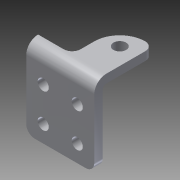
# Autodesk Inventor part: Clamp Piston Right Mount
Saved by Autodesk Inventor 2014 (Build 180170000, 170)
## iProperties
Created: 2014-02-22
Part Number: Clamp Piston Right Mount
Material: Aluminum 6061
Document SubType Name: Sheet Metal
Designer: Michael
Density: 1 g/cm^3
Sheet Metal Rule: Default
Appearance: Aluminum - Flat
Author: Michael
Autodesk Inventor part; units mm, degrees
ref_plane "YZ Plane" through (0, 0, 0) normal (1, 0, 0) x (0, 1, 0)
ref_plane "XZ Plane" through (0, 0, 0) normal (0, 1, 0) x (-1, 0, 0)
ref_plane "XY Plane" through (0, 0, 0) normal (0, 0, 1) x (1, 0, 0)
sketch "Sketch1" plane through (0, 0, 0) normal (0, 0, 1) x (1, 0, 0)
  line L0 (0, 0) -> (25.4, 0)
  line L1 (25.4, 0) -> (25.4, 25.4)
  line L2 (25.4, 25.4) -> (0, 25.4)
  line L3 (0, 25.4) -> (0, 0)
  circle A0 centre (6.35, 19.05) radius 2.0701
  circle A1 centre (19.05, 19.05) radius 2.0701
  circle A2 centre (6.35, 6.35) radius 2.0701
  circle A3 centre (19.05, 6.35) radius 2.0701
  dimension "d0" = 25.4
  dimension "d1" = 25.4
  dimension "d2" = 4.1402
  dimension "d3" = 6.35
  dimension "d4" = 6.35
  dimension "d7" = 12.7
  dimension "d10" = 12.7
  measures "d0" distance of L2.end L1.end
  measures "d1" distance of L1.end L0.end
  measures "d2" diameter of A0
  measures "d3" distance from line of L2 A0.centre
  measures "d4" distance from line of L3 A0.centre
  measures "d7" distance of A0.centre A1.centre
  measures "d10" distance of A0.centre A2.centre
extrude "Plate1" add sketch "Sketch1" along normal blind 3.175
sketch "Sketch2" plane through (25.4, 26.67, -1.27) normal (0, 1, 0) x (-1, 0, 0)
  line L0 (25.4, 0) -> (0, 0)
  line L1 (0, 0) -> (0, -17.78)
  line L2 (0, -17.78) -> (25.4, -17.78)
  line L3 (25.4, -17.78) -> (25.4, 0)
  constraints: 6 end point, 1 horizontal, 1 perpendicular, 1 vertical
edge flange "Flange1" height 22.225 angle 90 thickness 3.175 bend radius 1.27 thickness toward (0, 1, 0) relief straight relief width 3.175 relief depth 1.5875 edges at (12.7, 25.4, 0) wall of the first edge with corners at (0, 26.67, -1.27) (25.4, 26.67, -1.27) (25.4, 26.67, -19.05) (0, 26.67, -19.05)
bend "Bend1"
corner "Corner1"
sketch "Sketch3" plane through (0, 29.845, -19.05) normal (0, 1, 0) x (1, 0, 0)
  line L0 (0, -17.78) -> (25.4, -17.78) projected
  line L1 (25.4, 0) -> (25.4, -17.78) projected
  line L2 (0, 0) -> (25.4, 0) projected
  line L3 (0, -17.78) -> (0, 0) projected
  circle A0 centre (19.05, -6.35) radius 2.3749
  arc A1 (22.225, 0) -> (12.7, -9.525) centre (22.225, -9.525) ccw
  line L4 (12.7, -9.525) -> (12.7, -17.78)
  point P0 (0, -19.05)
  dimension "d24" = 4.7498
  dimension "d25" = 6.35
  dimension "d26" = 6.35
  dimension "d27" = 9.525
  dimension "d28" = 3.175
  constraints: 2 centre point, 2 end point, 2 point on circle, 2 tangent, 1 midpoint, 1 point on line
  measures "d24" diameter of A0
  measures "d25" distance from line of L1 A0.centre
  measures "d26" distance from line of L2 A0.centre
  measures "d27" radius of A1
  measures "d28" distance of L1.start A1.start
extrude "Extrusion1" cut sketch "Sketch3" against normal blind 25.4 contours L3 L2 A1 L4 L0 | A0
fillet "Fillet1" radius 3.175 4 edges at (12.7, 28.2575, -1.27) (0, 0, 1.5875) (25.4, 0, 1.5875) (25.4, 28.2575, -19.05)
equation "\"d14\" = BendReliefWidth"
equation "\"d15\" = BendReliefDepth"
equation "\"d16\" = MinimumRemnant"
equation "\"d17\" = BendRadius"
equation "\"d21\" = CornerReliefSize"
equation "\"d22\" = GapSize"
equation "\"d23\" = JacobiRadiusSize"
equation "\"BendRadius\" = Thickness"
equation "\"BendReliefWidth\" = Thickness"
equation "\"BendReliefDepth\" = 0.5 * Thickness"
equation "\"CornerReliefSize\" = 4 * Thickness"
equation "\"MinimumRemnant\" = 2 * Thickness"
equation "\"TransitionRadius\" = BendRadius"
equation "\"JacobiRadiusSize\" = BendRadius"
equation "\"GapSize\" = Thickness"
equation "\"d13\" = BendRadius"
equation "\"Thickness\" = 3.175"
body "Solid1"
